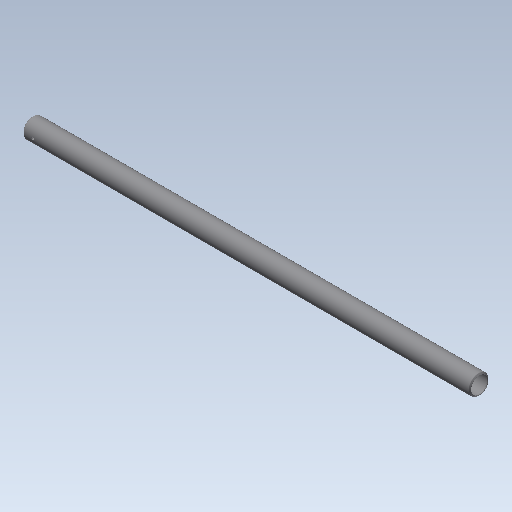
# Autodesk Inventor part: 01-10.8622
Saved by Autodesk Inventor 2020 (Build 240168000, 168)
## iProperties
Created: 2020-01-07
Part Number: 01-10.8622
Material: Generic
Catalog Web Link: www.cadenas.de
Description: Tube-Original Line - Standard Air Cylinders
Vendor: BIMBA
Document SubType Name: Modeling
Designer: psadmin
Manufacturer: BIMBA
Mass: 4.89669 g
Surface Area: 205.859 cm^2
Volume: 4.89669 cm^3
Density: 1 g/cm^3
Appearance: PSOLRGB-180-180-180
Category: PARTsolutions
Company: BIMBA
PSOL_IDENT_0: {$CADENAS_DATA\23d-libs\bimba\bimba_brand\bimba_imperial\bimba_full_line\original_line_cylinders\sta
PSOL_IDENT_1: ndard_air_cylinders\tube.prj},197 {VTYP=3D},{NB=01-10.8622},{LINA=01-10.8622},{NN=Tube},{DATE=23.12.
PSOL_IDENT_2: 2019 10:36:49},{GEOMDATE=18.02.2011 00:00:00},{VERSION=},{LINEID=20},{WBVAR=MNT,ACTING,NR,L,FOURHOLE
PSOL_IDENT_3: S,SR},{WBNUMERIC=L,FOURHOLES}  {NB=01-10.8622},{LINA=01-10.8622},{KT=DUMMY},{PN=01-10.8622},{BORE=0.
PSOL_IDENT_4: 43750000},{BOREPN=01},{MNT=},{MNTALG='' , 'Front Nose' , 'BF' , 'Front Block' , 'BFT' , 'Front Trunn
PSOL_IDENT_5: ion'},{ACTING=},{ACTINGALG= '' , 'Single Acting' , 'R' , 'Reverse/Double Acting' },{NR=},{NRALG= ''
PSOL_IDENT_6: , 'Without Non-rotating Rod' , 'NR' , 'With Non-rotating Rod' },{L=10.8620},{OD=0.4840},{ODN=0.4840}
PSOL_IDENT_7: ,{ODP=0.7380},{ODB=0.0000},{ID=0.4465},{DV=0.00000000},{LV=0.00000000},{LV1=0.00000000},{G=0.0200},{
PSOL_IDENT_8: FOURHOLES=2},{AA=0.2500},{BB=0.0620},{SR=},{SRALG= 'C' , 'Carbon Steel Rod' , 'SR' , '303 Stainless
PSOL_IDENT_9: Steel Rod' , '' , '303 Stainless Steel Rod'}
NN: Tube
NT: Original Line - Standard Air Cylinders
NB: 01-10.8622
NBSYN: $PN.
LINA: 01-10.8622
BORE: 0
BOREPN: 01
MNT: Front Nose
MNTALG: '' , 'Front Nose' , 'BF' , 'Front Block' , 'BFT' , 'Front Trunnion'
ACTING: Single Acting
NR: Without Non-rotating Rod
L: 10.862
ODN: 0.484
ODP: 0.738
ODB: 0
ID: 0.4465
DV: 0
LV: 0
LV1: 0
G: 0.02
FOURHOLES: 2
AA: 0.25
BB: 0.062
SR: 303 Stainless Steel Rod
SUPPLIER: BIMBA
ARTICLENO: 01-10.8622
BOMINFO: 01-10.8622
CREATOR: CADENAS GmbH
Title: 01-10.8622
Author: Cadenas PARTsolutions
Comments: Original Line - Standard Air Cylinders
Autodesk Inventor part; units mm, degrees
sketch "Sketch_1" plane through (0, 0, 0) normal (0, 0, 1) x (1, 0, 0)
  line L0 (275.8948, 0) -> (0, 0)
  arc A0 (-0.3964, 5.4846) -> (-0.3964, 5.305) centre (-0.3066, 5.3948) ccw
  line L1 (-0.3964, 5.305) -> (-0.254, 5.1626)
  line L2 (-0.254, 5.1626) -> (0, 5.1626)
  line L3 (0, 5.1626) -> (0.508, 5.6706)
  line L4 (0.508, 5.6706) -> (275.3868, 5.6706)
  line L5 (275.3868, 5.6706) -> (275.8948, 5.1626)
  line L6 (275.8948, 5.1626) -> (276.1488, 5.1626)
  line L7 (276.1488, 5.1626) -> (276.2912, 5.305)
  arc A1 (276.2912, 5.305) -> (276.2912, 5.4846) centre (276.2014, 5.3948) ccw
  line L8 (276.2912, 5.4846) -> (275.7778, 5.998)
  arc A2 (275.7778, 5.998) -> (275.4185, 6.1468) centre (275.4185, 5.6388) ccw
  line L9 (275.4185, 6.1468) -> (0.4763, 6.1468)
  arc A3 (0.4763, 6.1468) -> (0.117, 5.998) centre (0.4763, 5.6388) ccw
  line L10 (0.117, 5.998) -> (-0.3964, 5.4846)
  constraints: 22 end point, 8 point on circle, 4 centre point
revolve "Revolution1" add sketch "Sketch_1" angle 360 about axis through (275.8948, 0, 0) along (1, 0, 0)
sketch "Sketch_4" plane through (0, 0, 0) normal (0, 0, 1) x (1, 0, 0)
  circle A0 centre (5.842, 0) radius 0.7874
  constraints: 1 centre point
extrude "Extrusion1" cut sketch "Sketch_4" along normal blind 6.1468
ref_plane "cp1_XY" through (137.9474, 6.1468, 0) normal (1, 0, 0) x (0, 0, -1)
ref_plane "cp1_YZ" through (137.9474, 6.1468, 0) normal (0, 0, -1) x (0, 1, 0)
ref_plane "cp1_ZX" through (137.9474, 6.1468, 0) normal (0, 1, 0) x (1, 0, 0)
ref_plane "cp2_XY" through (137.9474, 0, -6.1468) normal (1, 0, 0) x (0, 0, -1)
ref_plane "cp2_YZ" through (137.9474, 0, -6.1468) normal (0, 0, -1) x (0, 1, 0)
ref_plane "cp2_ZX" through (137.9474, 0, -6.1468) normal (0, 1, 0) x (1, 0, 0)
ref_plane "cp3_XY" through (137.9474, -6.1468, 0) normal (1, 0, 0) x (0, 0, -1)
ref_plane "cp3_YZ" through (137.9474, -6.1468, 0) normal (0, 0, -1) x (0, 1, 0)
ref_plane "cp3_ZX" through (137.9474, -6.1468, 0) normal (0, 1, 0) x (1, 0, 0)
ref_plane "cp4_XY" through (137.9474, 0, 6.1468) normal (1, 0, 0) x (0, 0, -1)
ref_plane "cp4_YZ" through (137.9474, 0, 6.1468) normal (0, 0, -1) x (0, 1, 0)
ref_plane "cp4_ZX" through (137.9474, 0, 6.1468) normal (0, 1, 0) x (1, 0, 0)
ref_plane "tube_front_XY" through (0, 0, 0) normal (1, 0, 0) x (0, 0, -1)
ref_plane "tube_front_YZ" through (0, 0, 0) normal (0, 0, -1) x (0, 1, 0)
ref_plane "tube_front_ZX" through (0, 0, 0) normal (0, 1, 0) x (1, 0, 0)
ref_plane "tube_rear_XY" through (275.8948, 0, 0) normal (1, 0, 0) x (0, 0, -1)
ref_plane "tube_rear_YZ" through (275.8948, 0, 0) normal (0, 0, -1) x (0, 1, 0)
ref_plane "tube_rear_ZX" through (275.8948, 0, 0) normal (0, 1, 0) x (1, 0, 0)
body "Solid1"
